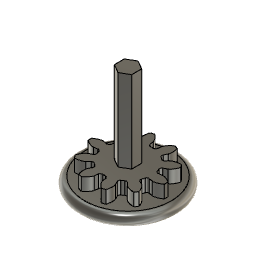
wheel left rear (Autodesk Fusion 360 design; units mm, degrees)
description: Spur Gear; Module: 2.2; Num Teeth: 10; Pressure Angle: 20.0; Backlash: 0.00 mm
Autodesk Fusion 360 part; units mm, degrees
sketch "wheel left rear 1" plane through (0, 0, 0) normal (0, 0, 1) x (1, 0, 0) in component "wheel left rear (1)"
  circle A0 centre (0, 0) radius 8.3092
  circle A1 centre (0, 0) radius 3.5
  circle A2 centre (0, 0) radius 17
  line L0 (-3.0019, 1.735) -> (0.0011, 3.4641)
  line L1 (0.0011, 3.4641) -> (2.9929, 1.735)
  line L2 (2.9929, 1.735) -> (3.0012, -1.7321)
  line L3 (3.0012, -1.7321) -> (0.0011, -3.4643)
  line L4 (0.0011, -3.4643) -> (-2.9989, -1.7321)
  line L5 (-2.9989, -1.7321) -> (-3.0019, 1.735)
  dimension "d195_1" = 7
  dimension "d196_1" = 34
  constraint coincident A0.centre A1.centre
  constraint concentric A1 A2
  measures "d195_1" diameter of A1
  measures "d196_1" diameter of A2
extrude "Extrude1" add sketch "wheel left rear 1" along normal blind 4.4 contours A0 | A1 | L0 L1 L2 L3 L4 L5 in component "wheel left rear (1)"
sketch "wheel left rear 2" plane through (0, 0, 0) normal (0, 0, 1) x (1, 0, 0) in component "wheel left rear (1)"
  spline S0 degree 5 poles (10.1841, -1.769) (10.1925, -1.7704) (10.2094, -1.7731) (10.2348, -1.7761) (10.2689, -1.7786) (10.3116, -1.7794) (10.3546, -1.7786) (10.3977, -1.7768) (10.4408, -1.7744) (10.484, -1.7717) (10.5273, -1.7685) (10.5706, -1.7648) (10.614, -1.7604) (10.6574, -1.7552) (10.7008, -1.7492) (10.7443, -1.7425) (10.7879, -1.7351) (10.8314, -1.7271) (10.875, -1.7187) (10.9186, -1.7098) (10.9622, -1.7005) (11.0058, -1.6907) (11.0494, -1.6804) (11.0931, -1.6695) (11.1367, -1.6581) (11.1803, -1.6463) (11.2239, -1.6339) (11.2675, -1.6212) (11.3111, -1.608) (11.3547, -1.5943) (11.3982, -1.5802) (11.4418, -1.5657) (11.4853, -1.5508) (11.5288, -1.5355) (11.5722, -1.5197) (11.6157, -1.5035) (11.6591, -1.4869) (11.7024, -1.4699) (11.7457, -1.4525) (11.789, -1.4347) (11.8323, -1.4166) (11.8755, -1.398) (11.9187, -1.3791) (11.9618, -1.3598) (12.0049, -1.3401) (12.0479, -1.32) (12.0909, -1.2996) (12.1338, -1.2787) (12.1766, -1.2576) (12.2194, -1.236) (12.2622, -1.2141) (12.3049, -1.1919) (12.3475, -1.1693) (12.3901, -1.1463) (12.4325, -1.123) (12.475, -1.0994) (12.5173, -1.0754) (12.5596, -1.0511) (12.6018, -1.0264) (12.6439, -1.0014) (12.686, -0.976) (12.728, -0.9503) (12.7699, -0.9243) (12.8117, -0.898) (12.8535, -0.8713) (12.8951, -0.8443) (12.9367, -0.817) (12.9782, -0.7893) (13.0195, -0.7613) (13.0608, -0.7331) (13.102, -0.7045) (13.1349, -0.6813) (13.1596, -0.6638) (13.176, -0.6521) (13.1842, -0.6462) knots 0 0 0 0 0 0 0.01428571 0.02857143 0.04285714 0.05714286 0.07142857 0.08571429 0.1 0.11428571 0.12857143 0.14285714 0.15714286 0.17142857 0.18571429 0.2 0.21428571 0.22857143 0.24285714 0.25714286 0.27142857 0.28571429 0.3 0.31428571 0.32857143 0.34285714 0.35714286 0.37142857 0.38571429 0.4 0.41428571 0.42857143 0.44285714 0.45714286 0.47142857 0.48571429 0.5 0.51428571 0.52857143 0.54285714 0.55714286 0.57142857 0.58571429 0.6 0.61428571 0.62857143 0.64285714 0.65714286 0.67142857 0.68571429 0.7 0.71428571 0.72857143 0.74285714 0.75714286 0.77142857 0.78571429 0.8 0.81428571 0.82857143 0.84285714 0.85714286 0.87142857 0.88571429 0.9 0.91428571 0.92857143 0.94285714 0.95714286 0.97142857 0.98571429 1 1 1 1 1 1
  spline S1 degree 5 poles (10.1841, 1.769) (10.1925, 1.7704) (10.2094, 1.7731) (10.2348, 1.7761) (10.2689, 1.7786) (10.3116, 1.7794) (10.3546, 1.7786) (10.3977, 1.7768) (10.4408, 1.7744) (10.484, 1.7717) (10.5273, 1.7685) (10.5706, 1.7648) (10.614, 1.7604) (10.6574, 1.7552) (10.7008, 1.7492) (10.7443, 1.7425) (10.7879, 1.7351) (10.8314, 1.7271) (10.875, 1.7187) (10.9186, 1.7098) (10.9622, 1.7005) (11.0058, 1.6907) (11.0494, 1.6804) (11.0931, 1.6695) (11.1367, 1.6581) (11.1803, 1.6463) (11.2239, 1.6339) (11.2675, 1.6212) (11.3111, 1.608) (11.3547, 1.5943) (11.3982, 1.5802) (11.4418, 1.5657) (11.4853, 1.5508) (11.5288, 1.5355) (11.5722, 1.5197) (11.6157, 1.5035) (11.6591, 1.4869) (11.7024, 1.4699) (11.7457, 1.4525) (11.789, 1.4347) (11.8323, 1.4166) (11.8755, 1.398) (11.9187, 1.3791) (11.9618, 1.3598) (12.0049, 1.3401) (12.0479, 1.32) (12.0909, 1.2996) (12.1338, 1.2787) (12.1766, 1.2576) (12.2194, 1.236) (12.2622, 1.2141) (12.3049, 1.1919) (12.3475, 1.1693) (12.3901, 1.1463) (12.4325, 1.123) (12.475, 1.0994) (12.5173, 1.0754) (12.5596, 1.0511) (12.6018, 1.0264) (12.6439, 1.0014) (12.686, 0.976) (12.728, 0.9503) (12.7699, 0.9243) (12.8117, 0.898) (12.8535, 0.8713) (12.8951, 0.8443) (12.9367, 0.817) (12.9782, 0.7893) (13.0195, 0.7613) (13.0608, 0.7331) (13.102, 0.7045) (13.1349, 0.6813) (13.1596, 0.6638) (13.176, 0.6521) (13.1842, 0.6462) knots 0 0 0 0 0 0 0.01428571 0.02857143 0.04285714 0.05714286 0.07142857 0.08571429 0.1 0.11428571 0.12857143 0.14285714 0.15714286 0.17142857 0.18571429 0.2 0.21428571 0.22857143 0.24285714 0.25714286 0.27142857 0.28571429 0.3 0.31428571 0.32857143 0.34285714 0.35714286 0.37142857 0.38571429 0.4 0.41428571 0.42857143 0.44285714 0.45714286 0.47142857 0.48571429 0.5 0.51428571 0.52857143 0.54285714 0.55714286 0.57142857 0.58571429 0.6 0.61428571 0.62857143 0.64285714 0.65714286 0.67142857 0.68571429 0.7 0.71428571 0.72857143 0.74285714 0.75714286 0.77142857 0.78571429 0.8 0.81428571 0.82857143 0.84285714 0.85714286 0.87142857 0.88571429 0.9 0.91428571 0.92857143 0.94285714 0.95714286 0.97142857 0.98571429 1 1 1 1 1 1
  arc A0 (13.1842, -0.6462) -> (13.1842, 0.6462) centre (0, 0) ccw
  line L0 (8.1768, -1.422) -> (10.1841, -1.769)
  line L1 (8.1768, 1.422) -> (10.1841, 1.769)
  line L2 (8.1768, -1.422) -> (8.1768, 1.422)
  point P0 (10.3903, -1.777)
  point P1 (10.6003, -1.7617)
  point P2 (10.8126, -1.7305)
  point P3 (11.0266, -1.6857)
  point P4 (11.2419, -1.6286)
  point P5 (11.4581, -1.5601)
  point P6 (11.6748, -1.4807)
  point P7 (11.8918, -1.3908)
  point P8 (12.1088, -1.2908)
  point P9 (12.3254, -1.1809)
  point P10 (12.5416, -1.0614)
  point P11 (12.7569, -0.9323)
  point P12 (12.9712, -0.7939)
  point P13 (10.3903, 1.777)
  point P14 (10.6003, 1.7617)
  point P15 (10.8126, 1.7305)
  point P16 (11.0266, 1.6857)
  point P17 (11.2419, 1.6286)
  point P18 (11.4581, 1.5601)
  point P19 (11.6748, 1.4807)
  point P20 (11.8918, 1.3908)
  point P21 (12.1088, 1.2908)
  point P22 (12.3254, 1.1809)
  point P23 (12.5416, 1.0614)
  point P24 (12.7569, 0.9323)
  point P25 (12.9712, 0.7939)
extrude "Extrude2" add sketch "wheel left rear 2" along normal blind 4.4 in component "wheel left rear (1)"
fillet "Fillet1" radius 0.75 2 edges at (8.1863, -1.4237, 2.2) (8.1863, 1.4237, 2.2) in component "wheel left rear (1)"
pattern_circular "C-Pattern1" count 10 over 360 about axis through (0, 0, 0) along (0, 0, 1) of "Extrude2", "Fillet1" in component "wheel left rear (1)"
sketch "wheel left rear 3" plane through (0, 0, 0) normal (0, 0, 1) x (1, 0, 0) in component "wheel left rear (1)"
  circle A0 centre (0, 0) radius 11 construction
mesh "Mesh1" [no effect] in component "wheel left rear (1)"
move_body "Move1" bodies 1 to x (1, 0, 0) y (0, 1, 0) z (0, 0, 1) at (0, 0, 12) in component "wheel left rear (1)"
move_body "Move2" bodies 1 to x (1, 0, 0) y (0, 1, 0) z (0, 0, 1) at (0, 0, -12) in component "wheel left rear (1)"
extrude "Extrude3" add sketch "wheel left rear 1" against normal blind 4 contours A0 | A1 | A2 | L0 L1 L2 L3 L4 L5 in component "wheel left rear (1)"
fillet "Fillet2" radius 2 2 edges at (-15.8496, -6.1475, 0) (-15.8496, 6.1475, -4) in component "wheel left rear (1)"
sketch "hexagon" plane through (0, 0, 0) normal (1, 0, 0) x (0, 1, 0) in component "wheel left rear (1)"
  line L0 (3.7184, 20.1371) -> (3.715, 48.525)
move_body "Move3" bodies 1 to x (1, 0, 0) y (0, 1, 0) z (0, 0, 1) at (0, 0, 4) in component "wheel left rear (1)"
extrude "Extrude4" add sketch "wheel left rear 1" along normal blind 36.738 contours L0 L1 L2 L3 L4 L5 in component "wheel left rear (1)"
move_body "Move4" bodies 1 to x (1, 0, 0) y (0, 1, 0) z (0, 0, 1) at (0, 0, 12) in component "wheel left rear (1)"
mesh "Mesh2" [no effect] in component "wheel left rear (1)"
mesh "Mesh3" [no effect] in component "wheel left rear (1)"
component "wheel left rear (1)" placed x (1, 0, 0) y (0, 1, 0) z (0, 0, 1) at (0, 0, 0)
equation "d201_1 = 4 mm + 4.4 mm + 28.338 mm"
named bodies: "wheel left rear"
